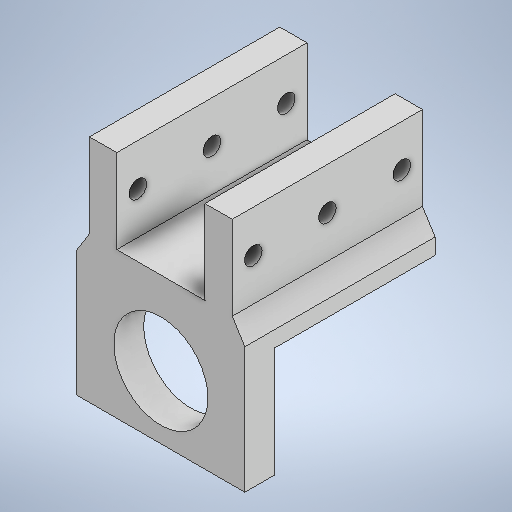
# Autodesk Inventor part: CH-4_DiffBarSupport
Saved by Autodesk Inventor 2025.1 (Build 291241000, 241)
## iProperties
Created: 2024-12-05
Part Number: CH-4_DiffBarSupport
Material: Generic
Document SubType Name: Modeling
Designer: aidan
Density: 1 g/cm^3
Appearance: Default
Author: aidan
Autodesk Inventor part; units mm, degrees
ref_plane "YZ Plane" through (0, 0, 0) normal (1, 0, 0) x (0, 1, 0)
ref_plane "XZ Plane" through (0, 0, 0) normal (0, 1, 0) x (-1, 0, 0)
ref_plane "XY Plane" through (0, 0, 0) normal (0, 0, 1) x (1, 0, 0)
sketch "Sketch1" plane through (0, 0, 0) normal (0, 0, 1) x (1, 0, 0)
  circle A0 centre (0, 0) radius 14.224
  line L0 (-25.4, -19.05) -> (25.4, -19.05)
  line L1 (25.4, -19.05) -> (25.4, 19.05)
  line L2 (25.4, 19.05) -> (-25.4, 19.05)
  line L3 (-25.4, 19.05) -> (-25.4, -19.05)
  line L4 (-25.4, -19.05) -> (25.4, 19.05) construction
  line L5 (25.4, -19.05) -> (-25.4, 19.05) construction
  line L6 (0, 0) -> (0, 25.146)
  line L7 (0, 25.146) -> (-12.7, 25.146)
  line L8 (-12.7, 25.146) -> (12.7, 25.146)
  line L9 (-12.7, 25.146) -> (-25.4, 19.05)
  line L10 (12.7, 25.146) -> (25.4, 19.05)
  line L11 (-12.7, 25.146) -> (-21.59, 25.146)
  line L12 (-21.59, 25.146) -> (-21.59, 50.546)
  line L13 (-21.59, 50.546) -> (-12.7, 50.546)
  line L14 (-12.7, 50.546) -> (-12.7, 25.146)
  line L15 (-21.59, 25.146) -> (-25.4, 19.05)
  line L16 (12.7, 25.146) -> (12.7, 50.546)
  line L17 (12.7, 50.546) -> (21.59, 50.546)
  line L18 (21.59, 50.546) -> (21.59, 25.146)
  line L19 (21.59, 25.146) -> (25.4, 19.05)
  line L20 (12.7, 25.146) -> (21.59, 25.146)
  dimension "d0" = 28.448
  dimension "d1" = 38.1
  dimension "d2" = 50.8
  dimension "d3" = 25.146
  dimension "d4" = 12.7
  dimension "d5" = 25.4
  dimension "d6" = 8.89
  dimension "d7" = 25.4
  dimension "d8" = 8.89
  constraints: 42 end point, 6 perpendicular, 3 horizontal, 3 parallel, 3 point on line, 2 midpoint, 1 centre point, 1 coincident, 1 vertical
  measures "d0" diameter of A0
  measures "d1" distance of L0.end L1.end
  measures "d2" distance of L1.end L2.end
  measures "d3" distance of L6.start L6.end
  measures "d4" distance of L6.end L7.end
  measures "d5" distance of L7.end L8.end
  measures "d6" distance of L7.end L11.end
  measures "d7" distance of L11.end L12.end
  measures "d8" distance of L16.end L17.end
extrude "Extrusion1" add sketch "Sketch1" along normal blind 6.7469
sketch "Sketch3" plane through (0, 0, 0) normal (0, 0, -1) x (-1, 0, 0)
  circle A0 centre (0, 0) radius 14.224
  line L0 (21.5903, 3.302) -> (-21.59, 3.302)
  line L1 (-21.59, 3.302) -> (-21.59, 25.146)
  line L2 (-21.59, 25.146) -> (21.5903, 25.146)
  line L3 (21.5903, 25.146) -> (21.5903, 3.302)
  circle A1 centre (0, 0) radius 14.224 projected
  line L4 (21.5903, 3.302) -> (-21.59, 25.146) construction
  line L5 (-21.59, 3.302) -> (21.5903, 25.146) construction
  line L6 (-25.4, -19.05) -> (-25.4, 19.05) projected
  line L7 (25.4, 19.05) -> (25.4, -19.05) projected
  line L8 (25.4, -19.05) -> (-25.4, -19.05) projected
  line L9 (25.4, 19.05) -> (25.4, -19.05) projected
  line L10 (21.59, 25.146) -> (25.4, 19.05) projected
  line L11 (21.59, 50.546) -> (21.59, 25.146) projected
  line L12 (12.7, 50.546) -> (21.59, 50.546) projected
  line L13 (12.7, 25.146) -> (12.7, 50.546) projected
  line L14 (-12.7, 25.146) -> (12.7, 25.146) projected
  line L15 (-12.7, 50.546) -> (-12.7, 25.146) projected
  line L16 (-21.59, 50.546) -> (-12.7, 50.546) projected
  line L17 (-21.59, 25.146) -> (-21.59, 50.546) projected
  line L18 (-25.4, 19.05) -> (-21.59, 25.146) projected
  line L19 (-25.4, -19.05) -> (-25.4, 19.05) projected
  circle A2 centre (0, 0) radius 14.224 projected
  line L20 (25.4, 3.302) -> (21.5903, 3.302)
  line L21 (-25.4, 3.302) -> (-21.59, 3.302)
  line L22 (0, 14.224) -> (-25.4, 14.224)
  point P0 (0.0002, 14.224)
  point P1 (-13.8354, 3.302)
  point P2 (13.8354, 3.302)
  dimension "d13" = 28.448
  constraints: 18 end point, 3 perpendicular, 3 point on line, 2 horizontal, 2 midpoint, 2 parallel, 1 coincident, 5 other
extrude "Extrusion3" add sketch "Sketch3" along normal blind 50.8 contours A0 L22 L1 L2 L3 L0 | L0 L1 L22 A0 | L3 L10 L7 L20 | L21 L6 L22 L1 | L22 L6 L18 L1 | L2 L13 L12 L11 | L17 L16 L15 L2
sketch "Sketch5" plane through (21.59, 50.546, 6.7469) normal (1, 0, 0) x (0, 0, -1)
  line L0 (57.5469, -25.4) -> (57.5469, 0) projected
  line L1 (0, -23.5788) -> (57.5469, -23.5788) projected
  line L2 (57.5469, 0) -> (57.5469, -23.5788)
  circle A0 centre (51.2625, -12.7) radius 2.6543
  line L3 (51.2625, -12.7) -> (57.5469, -11.7894)
  line L4 (57.5469, 0) -> (57.5469, -25.4) projected
  line L5 (57.5469, 0) -> (0, 0) projected
  line L6 (0, -25.4) -> (0, 0) projected
  line L7 (0, -12.7) -> (6.35, -12.7)
  circle A1 centre (6.35, -12.7) radius 2.6543
  circle A2 centre (28.7734, -12.7) radius 2.6543
  line L8 (6.35, -12.7) -> (28.7734, -12.7)
  line L9 (28.7734, -12.7) -> (51.2625, -12.7)
  line L10 (57.5469, -25.4) -> (0, -25.4) projected
  point P0 (6.7469, -50.546)
  dimension "d18" = 5.3086
  dimension "d19" = 6.35
  dimension "d20" = 6.35
  dimension "d21" = 5.3086
  dimension "d22" = 5.3086
  constraints: 10 end point, 3 centre point, 2 horizontal, 2 midpoint, 1 coincident, 1 collinear, 1 perpendicular
  measures "d18" diameter of A0
  measures "d19" distance of L3.start L3.end
  measures "d20" distance of L7.start L7.end
  measures "d21" diameter of A1
  measures "d22" diameter of A2
extrude "Extrusion4" cut sketch "Sketch5" against normal blind 133.35 contours L3 L9 A0 | A0 L9 L3 | A1 L8 L7 | L7 L8 A1 | L9 L8 A2 | A2 L8 L9
sketch "Sketch9" plane through (0, 0, -50.8) normal (0, 0, -1) x (-1, 0, 0)
  line L0 (-21.59, 50.546) -> (-12.7, 50.546) projected
  line L1 (13.335, -0.254) -> (-13.335, -0.254)
  line L2 (-13.335, -0.254) -> (-13.335, 50.546)
  line L3 (-13.335, 50.546) -> (13.335, 50.546)
  line L4 (13.335, 50.546) -> (13.335, -0.254)
  line L5 (-12.7, 25.146) -> (12.7, 25.146) projected
  line L6 (13.335, -0.254) -> (-13.335, 50.546) construction
  line L7 (-13.335, -0.254) -> (13.335, 50.546) construction
  line L8 (-25.4, -19.05) -> (-25.4, 19.05) projected
  line L9 (25.4, -19.05) -> (-25.4, -19.05)
  line L10 (-25.4, -19.05) -> (-25.4, 19.05)
  line L11 (-25.4, 19.05) -> (25.4, 19.05)
  line L12 (25.4, 19.05) -> (25.4, -19.05)
  line L13 (25.4, -19.05) -> (-25.4, 19.05) construction
  line L14 (-25.4, -19.05) -> (25.4, 19.05) construction
  point P0 (0, 0)
  point P1 (0, 25.146)
  point P2 (-13.335, 19.05)
  point P3 (13.335, 19.05)
  dimension "d27" = 26.67
  constraints: 24 end point, 5 midpoint, 4 parallel, 2 horizontal, 2 perpendicular, 1 point on line
  measures "d27" distance of L2.end L3.end
extrude "Extrusion5" cut sketch "Sketch9" against normal blind 42.8625
sketch "Sketch11" plane through (0, 0, 0) normal (0, 0, -1) x (-1, 0, 0)
  line L0 (25.4, 3.302) -> (13.8354, 3.302) projected
  arc A0 (-13.8354, 3.302) -> (13.8354, 3.302) centre (0, 0) ccw projected
  line L1 (-13.8354, 3.302) -> (-25.4, 3.302) projected
  line L2 (-25.4, -19.05) -> (-25.4, 3.302) projected
  line L3 (25.4, -19.05) -> (-25.4, -19.05) projected
  line L4 (25.4, 3.302) -> (25.4, -19.05) projected
  line L5 (12.7, 25.146) -> (12.7, 50.546) projected
  line L6 (-12.7, 25.146) -> (12.7, 25.146) projected
  line L7 (-12.7, 50.546) -> (-12.7, 25.146) projected
  line L8 (-13.335, 50.546) -> (-12.7, 50.546) projected
  line L9 (-13.335, 19.05) -> (-13.335, 50.546) projected
  line L10 (-25.4, 19.05) -> (-13.335, 19.05) projected
  line L11 (-25.4, 3.302) -> (-25.4, 19.05) projected
  line L12 (-13.8354, 3.302) -> (-25.4, 3.302) projected
  arc A1 (13.8354, 3.302) -> (-13.8354, 3.302) centre (0, 0) ccw projected
  line L13 (25.4, 3.302) -> (13.8354, 3.302) projected
  line L14 (25.4, 19.05) -> (25.4, 3.302) projected
  line L15 (13.335, 19.05) -> (25.4, 19.05) projected
  line L16 (13.335, 50.546) -> (13.335, 19.05) projected
  line L17 (12.7, 50.546) -> (13.335, 50.546) projected
extrude "Extrusion6" add sketch "Sketch11" along normal blind 2.286 contours L4 L3 L2 L1 A0 L0
sketch "Sketch12" plane through (0, 0, -7.9375) normal (0, 0, -1) x (-1, 0, 0)
  line L0 (12.7, 25.146) -> (12.7, 50.546) projected
  line L1 (-12.7, 25.146) -> (12.7, 25.146) projected
  line L2 (-12.7, 50.546) -> (-12.7, 25.146) projected
  line L3 (-13.335, 50.546) -> (-12.7, 50.546) projected
  line L4 (-13.335, 19.05) -> (-13.335, 50.546) projected
  line L5 (-25.4, 19.05) -> (-13.335, 19.05) projected
  line L6 (-25.4, 3.302) -> (-25.4, 19.05) projected
  line L7 (-13.8354, 3.302) -> (-25.4, 3.302) projected
  arc A0 (13.8354, 3.302) -> (-13.8354, 3.302) centre (0, 0) ccw projected
  line L8 (25.4, 3.302) -> (13.8354, 3.302) projected
  line L9 (25.4, 19.05) -> (25.4, 3.302) projected
  line L10 (13.335, 19.05) -> (25.4, 19.05) projected
  line L11 (13.335, 50.546) -> (13.335, 19.05) projected
  line L12 (12.7, 50.546) -> (13.335, 50.546) projected
extrude "Extrusion7" cut sketch "Sketch12" against normal blind 5.6515
sketch "Sketch13" plane through (0, 0, -2.286) normal (0, 0, -1) x (-1, 0, 0)
  line L0 (-12.7, 25.146) -> (12.7, 25.146) projected
  line L1 (-13.335, 19.05) -> (-13.335, 50.546) projected
  line L2 (12.7, 25.146) -> (-13.335, 25.146)
  line L3 (-13.335, 25.146) -> (-13.335, 50.546)
  line L4 (-13.335, 50.546) -> (12.7, 50.546)
  line L5 (12.7, 50.546) -> (12.7, 25.146)
  line L6 (13.335, 50.546) -> (13.335, 19.05) projected
  line L7 (12.7, 50.546) -> (13.335, 50.546)
  line L8 (13.335, 50.546) -> (13.335, 25.146)
  line L9 (13.335, 25.146) -> (12.7, 25.146)
  line L10 (12.7, 25.146) -> (12.7, 50.546)
  point P0 (0, 0)
  point P1 (-13.335, 25.146)
  constraints: 16 end point, 4 parallel, 2 horizontal, 2 perpendicular, 2 point on line
extrude "Extrusion8" cut sketch "Sketch13" against normal blind 37.211
sketch "Sketch14" plane through (0, 0, -2.286) normal (0, 0, -1) x (-1, 0, 0)
  circle A0 centre (0, 0) radius 14.224 projected
  line L0 (0, 14.224) -> (-25.4188, 14.224)
  line L1 (-25.4188, 14.224) -> (25.4, 14.224)
  line L2 (25.4, 19.05) -> (25.4, -19.05) projected
  line L3 (13.335, 25.146) -> (-13.335, 25.146) projected
  line L4 (-13.335, 19.05) -> (-13.335, 25.146) projected
  line L5 (-25.4, 19.05) -> (-13.335, 19.05) projected
  line L6 (-25.4, -19.05) -> (-25.4, 19.05) projected
  line L7 (-25.4, -19.05) -> (25.4, -19.05) projected
  line L8 (25.4, 19.05) -> (25.4, -19.05) projected
  line L9 (13.335, 19.05) -> (25.4, 19.05) projected
  line L10 (13.335, 25.146) -> (13.335, 19.05) projected
  circle A1 centre (0, 0) radius 14.224 projected
  line L11 (-13.335, 19.05) -> (-13.335, 50.546) projected
  line L12 (-13.335, 50.546) -> (-21.59, 50.546) projected
  line L13 (-21.59, 50.546) -> (-21.59, 25.146) projected
  line L14 (-21.59, 25.146) -> (-25.4, 19.05) projected
  line L15 (-25.4, 19.05) -> (-13.335, 19.05) projected
  line L16 (13.335, 50.546) -> (13.335, 19.05) projected
  line L17 (13.335, 19.05) -> (25.4, 19.05) projected
  line L18 (25.4, 19.05) -> (21.59, 25.146) projected
  line L19 (21.59, 25.146) -> (21.59, 50.546) projected
  line L20 (21.59, 50.546) -> (13.335, 50.546) projected
  line L21 (-21.59, 25.146) -> (21.59, 25.146)
  point P0 (-25.4, 14.224)
  constraints: 6 end point, 3 horizontal, 2 point on line, 1 vertical alignment, 1 other
extrude "Extrusion9" add sketch "Sketch14" along normal up to surface (48.514 mm away) contours L0 L6 L5 L4 L3 L10 L9 L2 L1 | L14 L21 L4 L5 | L9 L10 L21 L18
body "Solid1"
